Autodesk Fusion 360 part; units mm, degrees
(part 2 of 2)
  spline S15 degree 5 poles (25.9264, 40.0822) (25.9528, 40.123) (26.007, 40.2033) (26.0927, 40.3204) (26.2154, 40.4701) (26.3799, 40.6484) (26.5524, 40.8205) (26.7296, 40.989) (26.9092, 41.1554) (27.0907, 41.3204) (27.2742, 41.4836) (27.4604, 41.6444) (27.6501, 41.8022) (27.8437, 41.9565) (28.0411, 42.1074) (28.2419, 42.2552) (28.4454, 42.4004) (28.6513, 42.5433) (28.8591, 42.6841) (29.069, 42.823) (29.2808, 42.9596) (29.4948, 43.0941) (29.711, 43.2262) (29.9295, 43.3559) (30.1501, 43.4833) (30.3728, 43.6085) (30.5973, 43.7315) (30.8237, 43.8525) (31.0517, 43.9714) (31.2815, 44.0882) (31.513, 44.203) (31.7461, 44.3158) (31.9809, 44.4264) (32.2173, 44.5351) (32.4553, 44.6416) (32.6949, 44.7462) (32.936, 44.8487) (33.1785, 44.9493) (33.4225, 45.0479) (33.6679, 45.1445) (33.9146, 45.2392) (34.1627, 45.3319) (34.4122, 45.4227) (34.6629, 45.5115) (34.915, 45.5984) (35.1683, 45.6833) (35.4228, 45.7664) (35.6786, 45.8475) (35.9355, 45.9267) (36.1936, 46.004) (36.4528, 46.0794) (36.7132, 46.1529) (36.9746, 46.2245) (37.2372, 46.2942) (37.5008, 46.362) (37.7654, 46.428) (38.0311, 46.4921) (38.2977, 46.5543) (38.5654, 46.6146) (38.834, 46.6731) (39.1036, 46.7297) (39.3741, 46.7845) (39.6455, 46.8374) (39.9178, 46.8885) (40.191, 46.9377) (40.465, 46.985) (40.7399, 47.0305) (41.0156, 47.0742) (41.2922, 47.1161) (41.5695, 47.1561) (41.8476, 47.1942) (42.0707, 47.2233) (42.2384, 47.2443) (42.3504, 47.2579) (42.4064, 47.2647) knots 0 0 0 0 0 0 0.01428571 0.02857143 0.04285714 0.05714286 0.07142857 0.08571429 0.1 0.11428571 0.12857143 0.14285714 0.15714286 0.17142857 0.18571429 0.2 0.21428571 0.22857143 0.24285714 0.25714286 0.27142857 0.28571429 0.3 0.31428571 0.32857143 0.34285714 0.35714286 0.37142857 0.38571429 0.4 0.41428571 0.42857143 0.44285714 0.45714286 0.47142857 0.48571429 0.5 0.51428571 0.52857143 0.54285714 0.55714286 0.57142857 0.58571429 0.6 0.61428571 0.62857143 0.64285714 0.65714286 0.67142857 0.68571429 0.7 0.71428571 0.72857143 0.74285714 0.75714286 0.77142857 0.78571429 0.8 0.81428571 0.82857143 0.84285714 0.85714286 0.87142857 0.88571429 0.9 0.91428571 0.92857143 0.94285714 0.95714286 0.97142857 0.98571429 1 1 1 1 1 1
  line L15 (25.9264, 40.0822) -> (20.1277, 31.1207)
  arc A31 (17.9906, 30.6144) -> (20.1277, 31.1207) centre (18.7949, 31.9831) ccw
  arc A32 (17.9906, 30.6144) -> (8.9264, 34.3689) centre (0, 0) ccw
  circle A33 centre (0, 0) radius 7
  circle A34 centre (0, 0) radius 10
  line L16 (0, 13) -> (0, -12)
  circle A35 centre (0, 0) radius 27.5
  circle A36 centre (0, 0) radius 15
  line L17 (0, 0) -> (-5.1303, 14.0954)
  line L18 (0, 0) -> (5.1303, 14.0954)
  line L19 (-5.1303, 14.0954) -> (-9.4056, 25.8415)
  line L20 (5.1303, 14.0954) -> (9.4056, 25.8415)
  line L21 (-14.7721, 2.6047) -> (-27.0822, 4.7753)
  line L22 (-9.6418, 11.4907) -> (-17.6767, 21.0662)
  line L23 (-9.6418, -11.4907) -> (-17.6767, -21.0662)
  line L24 (-14.7721, -2.6047) -> (-27.0822, -4.7753)
  line L25 (5.1303, -14.0954) -> (9.4056, -25.8415)
  line L26 (-5.1303, -14.0954) -> (-9.4056, -25.8415)
  line L27 (14.7721, -2.6047) -> (27.0822, -4.7753)
  line L28 (9.6418, -11.4907) -> (17.6767, -21.0662)
  line L29 (9.6418, 11.4907) -> (17.6767, 21.0662)
  line L30 (14.7721, 2.6047) -> (27.0822, 4.7753)
  point P0 (0, 7)
  dimension "d25" = 14
  dimension "d30" = 3
  dimension "d37" = 55
  dimension "d38" = 30
  dimension "d39" = 40
  dimension "d40" = 20
  dimension "d42" = 360
  constraint concentric A0 A33
  constraint vertical L16
  constraint coincident A0.centre L16
  constraint coincident L16 P0
  constraint coincident A33 P0
  constraint concentric A33 A35
  constraint concentric A33 A36
  constraint coincident A0.centre A2.centre
  constraint coincident A35 L19.end
  constraint coincident A35 L20.end
  constraint coincident A36 L17.end
  constraint coincident A36 L18.end
  measures "d25" diameter of A33
  measures "d37" diameter of A35
  measures "d38" diameter of A36
  measures "d39" angle of L17 L18
  measures "d40" angle of L16 L18
extrude "Extrude3" cut sketch "Sketch1 (3)" against normal up to surface (32.7 mm away) contours A0 A33 L16 L18 | A0 A33 L16 L18 | A0 A33 L16 L17 | A0 A33 L16 L17 bodies 1 in component "Spur Gear (8 teeth)"
extrude "Extrude3'" cut sketch "Sketch1 (3)" against normal up to surface (32.7 mm away) contours A0 A33 L16 L18 | A0 A33 L16 L18 | A0 A33 L16 L17 | A0 A33 L16 L17 bodies 2 in component "Spur Gear (4 teeth)"
extrude "Extrude4" add sketch "Sketch1 (3)" against normal up to surface (32.7 mm away) contours A33 A34 L16 L18 | A33 A34 L16 L18 | A33 A34 L16 L17 | A33 A34 L16 L17 bodies 1 in component "Spur Gear (8 teeth)"
extrude "Extrude6" cut sketch "Sketch1 (3)" against normal up to surface (12.7 mm away) contours A35 A36 L19 L20 | A35 A36 L29 L30 | A35 A36 L21 L22 | A35 A36 L27 L28 | A35 A36 L23 L24 | A35 A36 L25 L26 bodies 1 in component "Spur Gear (8 teeth)"
component "Spur Gear (8 teeth)" placed x (1, 0, 0) y (0, 1, 0) z (0, 0, 1) at (0, 0, 0)
component "Spur Gear (4 teeth)" placed x (1, 0, 0) y (0, 1, 0) z (0, 0, 1) at (0, 0, 0)
